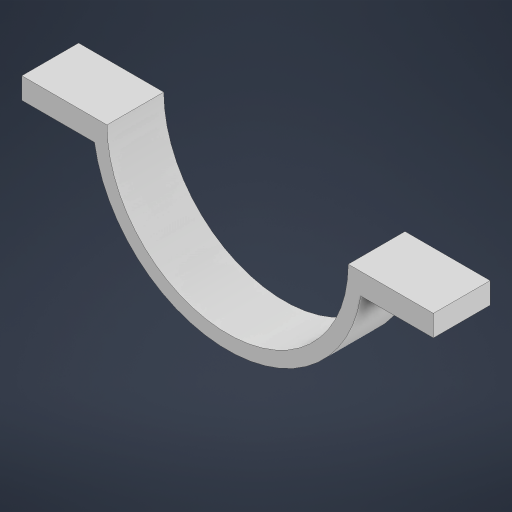
# Autodesk Inventor part: Part3
Saved by Autodesk Inventor 2023 (Build 270158030, 158C)
## iProperties
Created: 2023-02-03
Part Number: Part3
Material: Generic
Document SubType Name: Modeling
Designer: Monster
Density: 1 g/cm^3
Appearance: Default
Author: Monster
Autodesk Inventor part; units mm, degrees
ref_plane "YZ Plane" through (0, 0, 0) normal (1, 0, 0) x (0, 1, 0)
ref_plane "XZ Plane" through (0, 0, 0) normal (0, 1, 0) x (-1, 0, 0)
ref_plane "XY Plane" through (0, 0, 0) normal (0, 0, 1) x (1, 0, 0)
sketch "Sketch2" plane through (0, 0, 0) normal (0, 0, 1) x (1, 0, 0)
  arc A0 (-4.25, 0) -> (4.25, 0) centre (0, 0) ccw
  line L0 (4.25, 0) -> (7.25, 0)
  line L1 (-4.25, 0) -> (-7.25, 0)
  arc A1 (-4.6904, -0.75) -> (4.6904, -0.75) centre (0, 0) ccw
  line L2 (-7.25, 0) -> (-7.25, -0.75)
  line L3 (-7.25, -0.75) -> (-4.6904, -0.75)
  line L4 (7.25, 0) -> (7.25, -0.75)
  line L5 (7.25, -0.75) -> (4.6904, -0.75)
  dimension "d8" = 8.5
  dimension "d9" = 3
  dimension "d10" = 3
  dimension "d11" = 9.5
  dimension "d12" = 0.75
  constraints: 12 end point, 4 point on circle, 2 centre point, 2 coincident, 2 horizontal, 2 perpendicular, 2 point on line, 1 vertical
  measures "d8" diameter of A0
  measures "d9" distance of L0.start L0.end
  measures "d10" distance of L1.start L1.end
  measures "d11" diameter of A1
  measures "d12" distance of L1.end L2.end
extrude "Extrusion2" add sketch "Sketch2" along normal blind 2
body "Solid2"
